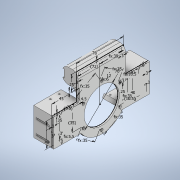
# Autodesk Inventor part: 6boltpaddles
Saved by Autodesk Inventor 2020.3 (Build 243373000, 373)
## iProperties
Created: 2020-09-18
Part Number: 6boltpaddles
Material: Generic
Document SubType Name: Modeling
Designer: joesp
Density: 1 g/cm^3
Appearance: Default
Author: joesp
Autodesk Inventor part; units mm, degrees
ref_plane "YZ Plane" through (0, 0, 0) normal (1, 0, 0) x (0, 1, 0)
ref_plane "XZ Plane" through (0, 0, 0) normal (0, 1, 0) x (-1, 0, 0)
ref_plane "XY Plane" through (0, 0, 0) normal (0, 0, 1) x (1, 0, 0)
sketch "Sketch1" plane through (0, 0, 0) normal (1, 0, 0) x (0, 1, 0)
  circle A0 centre (0, 0) radius 35 construction
  circle A1 centre (35, 0) radius 2.25
  circle A2 centre (-35, 0) radius 2.25
  circle A3 centre (17.5, -30.3109) radius 2.25
  circle A4 centre (-17.5, -30.3109) radius 2.25
  circle A5 centre (17.5, 30.3109) radius 2.25
  circle A6 centre (-17.5, 30.3109) radius 2.25
  circle A7 centre (0, 0) radius 29
  circle A8 centre (0, 0) radius 41
  line L0 (23, -33.9411) -> (-23, -33.9411)
  line L1 (-23, -33.9411) -> (-23, -78.9411)
  line L2 (-23, -78.9411) -> (23, -78.9411)
  line L3 (23, -78.9411) -> (23, -33.9411)
  line L4 (23, 33.9411) -> (-23, 33.9411)
  line L5 (-23, 33.9411) -> (-23, 78.9411)
  line L6 (-23, 78.9411) -> (23, 78.9411)
  line L7 (23, 78.9411) -> (23, 33.9411)
  line L8 (20, -75.9411) -> (-20, -75.9411) construction
  line L9 (-20, -75.9411) -> (-20, -65.9411) construction
  line L10 (-20, -65.9411) -> (20, -65.9411) construction
  line L11 (20, -65.9411) -> (20, -75.9411) construction
  line L12 (20, 65.9411) -> (-20, 65.9411) construction
  line L13 (-20, 65.9411) -> (-20, 75.9411) construction
  line L14 (-20, 75.9411) -> (20, 75.9411) construction
  line L15 (20, 75.9411) -> (20, 65.9411) construction
  line L16 (66, 39) -> (41, 39)
  line L17 (41, 39) -> (41, -39)
  line L18 (41, -39) -> (66, -39)
  line L19 (66, -39) -> (66, 39)
  line L20 (41, 39) -> (12.6491, 39)
  line L21 (41, -39) -> (12.6491, -39)
  line L22 (12.5, -42.9411) -> (-12.5, -42.9411) construction
  line L23 (-12.5, -42.9411) -> (-12.5, -62.9411) construction
  line L24 (-12.5, -62.9411) -> (12.5, -62.9411) construction
  line L25 (12.5, -62.9411) -> (12.5, -42.9411) construction
  line L26 (17.5, 62.9411) -> (-17.5, 62.9411) construction
  line L27 (-17.5, 62.9411) -> (-17.5, 42.9411) construction
  line L28 (-17.5, 42.9411) -> (17.5, 42.9411) construction
  line L29 (17.5, 42.9411) -> (17.5, 62.9411) construction
  line L30 (20, 75.9411) -> (-20, 75.9411)
  line L31 (-20, 75.9411) -> (-20, 35.7911)
  line L32 (-20, 35.7911) -> (20, 35.7911)
  line L33 (20, 35.7911) -> (20, 75.9411)
  line L34 (63, -36) -> (44, -36)
  line L35 (44, -36) -> (44, 36)
  line L36 (44, 36) -> (63, 36)
  line L37 (63, 36) -> (63, -36)
  line L38 (20, -75.9411) -> (-20, -75.9411)
  line L39 (-20, -75.9411) -> (-20, -36.9411)
  line L40 (-20, -36.9411) -> (20, -36.9411)
  line L41 (20, -36.9411) -> (20, -75.9411)
  point P0 (0, 75.9411)
  point P1 (0, 78.9411)
  point P2 (0, -75.9411)
  point P3 (0, -78.9411)
  point P4 (23, -39)
  point P5 (23, 39)
  point P6 (17.7863, -36.9411)
  point P7 (-17.7863, -36.9411)
  point P8 (-20, 35.7911)
  dimension "d0" = 70
  dimension "d1" = 35
  dimension "d2" = 35
  dimension "d3" = 35
  dimension "d4" = 35
  dimension "d5" = 35
  dimension "d6" = 35
  dimension "d7" = 4.5
  dimension "d8" = 12
  dimension "d9" = 6
  dimension "d10" = 10
  dimension "d11" = 40
  dimension "d12" = 10
  dimension "d13" = 40
  dimension "d14" = 78
  dimension "d15" = 25
  dimension "d16" = 39
  dimension "d17" = 25
  dimension "d18" = 20
  dimension "d19" = 35
  dimension "d20" = 20
  dimension "d23" = 3
  dimension "d24" = 3
  dimension "d25" = 45
  dimension "d26" = 3
  dimension "d27" = 10.5
  dimension "d28" = 10.5
  dimension "d29" = 3
  dimension "d31" = 5.5
  dimension "d32" = 3
  dimension "d34" = 5.5
  dimension "d37" = 3
  dimension "d40" = 3
  dimension "d41" = 3
  dimension "d42" = 3
  dimension "d43" = 3
  dimension "d44" = 3
  dimension "d45" = 72
  dimension "d46" = 3
  dimension "d47" = 3
  dimension "d48" = 3
  dimension "d49" = 3
  dimension "d50" = 3
  constraints: 84 end point, 21 parallel, 12 point on circle, 11 horizontal, 10 perpendicular, 9 centre point, 5 equal radius, 4 coincident, 4 midpoint, 2 point on line, 2 vertical alignment, 1 collinear, 1 horizontal alignment, 1 tangent
  measures "d0" diameter of A0
  measures "d1" distance of A1.centre A5.centre
  measures "d2" distance of A3.centre A1.centre
  measures "d3" distance of A4.centre A3.centre
  measures "d4" distance of A2.centre A4.centre
  measures "d5" distance of A6.centre A2.centre
  measures "d6" distance of A5.centre A6.centre
  measures "d7" diameter of A5
  measures "d8" radial gap between concentric circles of A8 A7
  measures "d9" radial gap between concentric circles of A0 A7
  measures "d10" distance of L10.end L8.start
  measures "d11" distance of L9.end L10.end
  measures "d12" distance of L14.end L12.start
  measures "d13" distance of L14.start L14.end
  measures "d14" distance of L18.end L16.start
  measures "d15" distance of L16.start L16.end
  measures "d16" distance from line of point (0, 0) L18
  measures "d17" distance of L22.start L22.end
  measures "d18" distance of L24.end L22.start
  measures "d19" distance of L26.start L26.end
  measures "d20" distance of L28.end L26.start
  measures "d23" distance between parallel lines of L26 L12
  measures "d24" distance between parallel lines of L6 L14
  measures "d25" distance of L6.end L4.start
  measures "d26" distance between parallel lines of L10 L24
  measures "d27" distance between parallel lines of L3 L25
  measures "d28" distance between parallel lines of L1 L23
  measures "d29" distance between parallel lines of L2 L8
  measures "d31" distance between parallel lines of L5 L27
  measures "d32" distance between parallel lines of L7 L15
  measures "d34" distance between parallel lines of L7 L29
  measures "d37" distance between parallel lines of L6 L30
  measures "d40" distance between parallel lines of L33 L7
  measures "d41" distance between parallel lines of L5 L31
  measures "d42" distance between parallel lines of L16 L36
  measures "d43" distance between parallel lines of L19 L37
  measures "d44" distance between parallel lines of L18 L34
  measures "d45" distance of L36.end L34.start
  measures "d46" distance between parallel lines of L17 L35
  measures "d47" distance between parallel lines of L1 L39
  measures "d48" distance between parallel lines of L2 L38
  measures "d49" distance between parallel lines of L3 L41
  measures "d50" distance between parallel lines of L0 L40
extrude "Extrusion1" add sketch "Sketch1" along normal blind 3 contours A8 L0 L4 | L17 L21 L3 A8 | A8 L7 L20 L17 | L17 L16 L19 L18 | L4 A8 L32 | A8 L33 L20 L7 | L3 L21 L41 L40 A8 | A8 L40 L0 | L32 A8 | A8 L20 L33 | L5 L6 L7 L20 L33 L30 L31 A8 | L40 L41 L21 A8 | A8 L40 | A8 L40 L39 L38 L41 L21 L3 L2 L1 | A8 L31 L30 L33 L20 | L21 L41 L38 L39 L40 A8 | L34 L35 L36 L37
extrude "Extrusion2" add sketch "Sketch1" against normal blind 30 contours A8 L33 L20 L7 | L3 L21 L41 L40 A8 | L5 L6 L7 L20 L33 L30 L31 A8 | A8 L40 L39 L38 L41 L21 L3 L2 L1
extrude "Extrusion3" add sketch "Sketch1" against normal blind 20 contours L17 L16 L19 L18
fillet "Fillet1" radius 9 3 edges at (3, 66, 0) (0, 63, 0) (0, 44, 0)
sketch "Sketch3" plane through (-20, 0, 0) normal (-1, 0, 0) x (0, 0, 1)
  line L0 (39, 66) -> (39, 57) projected
  line L1 (-39, 57) -> (-39, 66) projected
  line L2 (39, 66) -> (-39, 66)
  line L3 (-39, 66) -> (-39, 60)
  line L4 (-39, 60) -> (39, 60)
  line L5 (39, 60) -> (39, 66)
  line L6 (-39, 66) -> (-39, 41) projected
  line L7 (-39, 41) -> (39, 41)
  line L8 (39, 41) -> (39, 47)
  line L9 (39, 47) -> (-39, 47)
  line L10 (-39, 47) -> (-39, 41)
  line L11 (-39, 66) -> (39, 66) projected
  line L12 (10, 66) -> (10, 60)
  line L13 (10, 47) -> (10, 41)
  line L14 (39, 41) -> (-39, 41) projected
  line L15 (-10, 66) -> (-10, 60)
  line L16 (-10, 47) -> (-10, 41)
  line L17 (-33, 66) -> (-33, 60)
  line L18 (-33, 47) -> (-33, 41)
  line L19 (33, 66) -> (33, 60)
  line L20 (33, 47) -> (33, 41)
  line L21 (-39, 41) -> (39, 41) projected
  point P0 (0, 0)
  dimension "d58" = 6
  dimension "d59" = 6
  dimension "d62" = 20
  dimension "d63" = 6
  dimension "d64" = 6
  dimension "d65" = 29
  dimension "d66" = 29
  constraints: 32 end point, 26 point on line, 5 perpendicular, 4 parallel, 2 horizontal, 1 vertical
  measures "d58" distance of L7.end L8.end
  measures "d59" distance between parallel lines of L2 L4
  measures "d62" distance between parallel lines of L15 L12
  measures "d63" distance between parallel lines of L5 L19
  measures "d64" distance between parallel lines of L1 L17
  measures "d65" distance between parallel lines of L0 L12
  measures "d66" distance between parallel lines of L6 L15
extrude "Extrusion4" add sketch "Sketch3" along normal blind 2 contours L0 L4 L19 L2 | L12 L4 L15 L2 | L17 L4 L1 L2 | L9 L18 L7 L6 | L9 L13 L7 L16 | L9 L8 L7 L20
fillet "Fillet3" radius 10 12 edges at (-20, 63, 0) (-20, 63, -34.5) (-20, 44, -34.5) (-20, 44, 0) (-20, 44, 34.5) (-20, 63, 34.5) (-22, 66, 36) (-22, 66, 0) (-22, 66, -36) (-22, 41, 0) (-22, 41, 36) (-22, 41, -36)
chamfer "Chamfer1" distance 5 angle 45 1 edges at (0, 41, 0)
extrude "Extrusion5" cut sketch "Sketch1" against normal through all contours A8 L0 L4
sketch "Sketch4" plane through (3, -23, -78.9411) normal (0, -1, 0) x (1, 0, 0)
  circle A0 centre (-28, 22.5) radius 1.25
  circle A1 centre (-28, 135.3823) radius 1.25
  line L0 (-33, 112.8823) -> (-33, 157.8823) projected
  line L1 (-33, 157.8823) -> (0, 157.8823) projected
  line L2 (-3, 112.8823) -> (-33, 112.8823) projected
  line L3 (-3, 45) -> (-33, 45) projected
  line L4 (-33, 0) -> (0, 0) projected
  line L5 (-33, 0) -> (-33, 45) projected
  circle A2 centre (-28, 120.8823) radius 1.25
  circle A3 centre (-28, 37) radius 1.25
  point P0 (-3, 78.9411)
  dimension "d73" = 2.5
  dimension "d74" = 2.5
  dimension "d75" = 5
  dimension "d76" = 22.5
  dimension "d77" = 22.5
  dimension "d78" = 22.5
  dimension "d79" = 22.5
  dimension "d80" = 5
  dimension "d83" = 2.5
  dimension "d84" = 8
  dimension "d85" = 2.5
  dimension "d86" = 8
  constraints: 4 centre point, 2 vertical alignment
  measures "d73" diameter of A1
  measures "d74" diameter of A0
  measures "d75" distance from line of L0 A1.centre
  measures "d76" distance from line of L1 A1.centre
  measures "d77" distance from line of L2 A1.centre
  measures "d78" distance from line of L3 A0.centre
  measures "d79" distance from line of L4 A0.centre
  measures "d80" distance from line of L5 A0.centre
  measures "d83" diameter of A2
  measures "d84" distance from line of L2 A2.centre
  measures "d85" diameter of A3
  measures "d86" distance from line of L3 A3.centre
extrude "Extrusion6" cut sketch "Sketch4" against normal through all
sketch "Sketch5" plane through (3, -23, 78.9411) normal (0, 0, 1) x (1, 0, 0)
  line L0 (-28, 6.5) -> (-8, 6.5) construction
  line L1 (-28, 5.25) -> (-8, 5.25)
  line L2 (-8, 7.75) -> (-28, 7.75)
  arc A0 (-28, 7.75) -> (-28, 5.25) centre (-28, 6.5) ccw
  arc A1 (-8, 5.25) -> (-8, 7.75) centre (-8, 6.5) ccw
  line L3 (-28, 29.5) -> (-8, 29.5) construction
  line L4 (-28, 30.75) -> (-8, 30.75)
  line L5 (-8, 28.25) -> (-28, 28.25)
  arc A2 (-28, 30.75) -> (-28, 28.25) centre (-28, 29.5) ccw
  arc A3 (-8, 28.25) -> (-8, 30.75) centre (-8, 29.5) ccw
  line L6 (-3, 3) -> (-33, 3) projected
  line L7 (-33, 0) -> (-33, 46) projected
  line L8 (-3, 3) -> (-3, 43) projected
  point P0 (-3, 23)
  point P1 (-18, 6.5)
  point P2 (-18, 29.5)
  dimension "d87" = 23
  dimension "d88" = 3.5
  dimension "d89" = 2.5
  dimension "d90" = 2.5
  dimension "d91" = 5
  dimension "d92" = 5
  constraints: 16 end point, 8 point on circle, 8 tangent, 4 centre point, 3 parallel, 2 midpoint, 2 vertical alignment, 1 horizontal
  measures "d87" distance between parallel lines of L3 L0
  measures "d88" distance between parallel lines of L6 L0
  measures "d89" distance between parallel lines of L2 L1
  measures "d90" distance between parallel lines of L4 L5
  measures "d91" distance from line of L7 L0.start
  measures "d92" distance from line of L8 L0.end
extrude "Extrusion7" cut sketch "Sketch5" against normal through all
equation "\"d1\" = d6"
equation "\"d2\" = d6"
equation "\"d3\" = d6"
equation "\"d4\" = d6"
equation "\"d5\" = d6"
equation "\"d9\" = 0.5 * d8"
equation "\"d16\" = 0.5 * d14"
equation "\"d27\" = d28"
equation "\"d31\" = d34"
body "Solid1"
